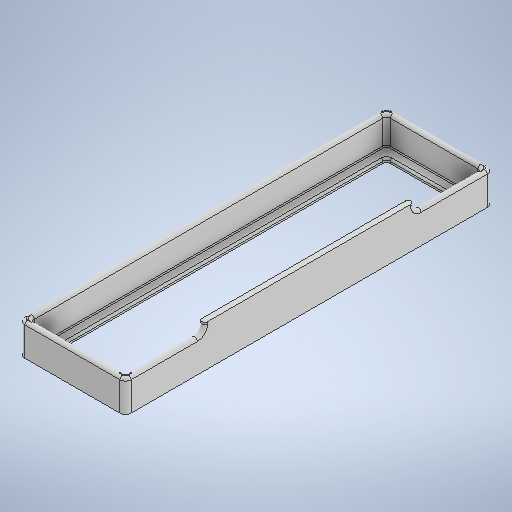
# Autodesk Inventor part: Case for ToolBox
Saved by Autodesk Inventor 2025 (Build 290162000, 162)
## iProperties
Created: 2024-11-06
Part Number: Case for ToolBox
Material: Типовые
Document SubType Name: Modeling
Designer: Makusimu
Density: 1 g/cm^3
Appearance: По умолчанию
Author: Makusimu
Autodesk Inventor part; units mm, degrees
ref_plane "YZ Plane" through (0, 0, 0) normal (1, 0, 0) x (0, 1, 0)
ref_plane "XZ Plane" through (0, 0, 0) normal (0, 1, 0) x (-1, 0, 0)
ref_plane "XY Plane" through (0, 0, 0) normal (0, 0, 1) x (1, 0, 0)
sketch "Эскиз1" plane through (0, 0, 0) normal (0, 1, 0) x (-1, 0, 0)
  line L0 (0, 0) -> (57, 0)
  line L1 (57, 0) -> (57, -197)
  line L2 (57, -197) -> (0, -197)
  line L3 (0, -197) -> (0, 0)
  line L4 (48.5, -8.5) -> (8.5, -8.5)
  line L5 (8.5, -8.5) -> (8.5, -188.5)
  line L6 (8.5, -188.5) -> (48.5, -188.5)
  line L7 (48.5, -188.5) -> (48.5, -8.5)
  point P0 (48.5, -98.5)
  point P1 (57, -98.5)
  point P2 (28.5, 0)
  point P3 (28.5, -8.5)
  dimension "d0" = 57
  dimension "d1" = 197
  dimension "d2" = 40
  dimension "d3" = 180
  dimension "d4" = 0
  dimension "d5" = 0
  constraints: 16 end point, 4 midpoint, 4 parallel, 2 horizontal, 2 perpendicular
  measures "d0" distance of L1.end L2.end
  measures "d1" distance of L0.end L1.end
  measures "d2" distance of L6.end L5.end
  measures "d3" distance of L5.end L4.end
  measures "d4" vertical distance of point (48.5, -98.5) point (57, -98.5)
  measures "d5" horizontal distance of point (28.5, 0) point (28.5, -8.5)
extrude "Выдавливание1" add sketch "Эскиз1" along normal blind 2
sketch "Эскиз2" plane through (0, 2, 0) normal (0, 1, 0) x (1, 0, 0)
  line L0 (-54, 3) -> (-3, 3)
  line L1 (-3, 3) -> (-3, 194)
  line L2 (-3, 194) -> (-54, 194)
  line L3 (-54, 194) -> (-54, 3)
  line L4 (-57, 197) -> (-57, 0) projected
  line L5 (-57, 0) -> (0, 0) projected
  line L6 (0, 0) -> (0, 197) projected
  line L7 (-57, 0) -> (0, 0)
  line L8 (0, 0) -> (0, 197)
  line L9 (0, 197) -> (-57, 197)
  line L10 (-57, 197) -> (-57, 0)
  point P0 (-57, 98.5)
  point P1 (-54, 98.5)
  point P2 (-28.5, 0)
  point P3 (-28.5, 3)
  dimension "d8" = 51
  dimension "d9" = 191
  dimension "d10" = 0
  dimension "d11" = 0
  constraints: 16 end point, 4 midpoint, 4 parallel, 2 horizontal, 2 perpendicular
  measures "d8" distance of L2.end L1.end
  measures "d9" distance of L1.end L0.end
  measures "d10" vertical distance of point (-57, 98.5) point (-54, 98.5)
  measures "d11" horizontal distance of point (-28.5, 0) point (-28.5, 3)
extrude "Выдавливание2" add sketch "Эскиз2" along normal blind 15
fillet "Сопряжение1" radius 2 4 edges at (-48.5, 1, -188.5) (-8.5, 1, -8.5) (-8.5, 1, -188.5) (-48.5, 1, -8.5)
fillet "Сопряжение2" radius 2 4 edges at (-54, 9.5, -3) (-3, 9.5, -3) (-3, 9.5, -194) (-54, 9.5, -194)
fillet "Сопряжение3" radius 3 4 edges at (0, 8.5, 0) (-57, 8.5, 0) (0, 8.5, -197) (-57, 8.5, -197)
fillet "Сопряжение5" radius 0.5 8 edges at (-3.5858, 2, -193.4142) (-28.5, 2, -194) (-53.4142, 2, -193.4142) (-54, 2, -98.5) (-53.4142, 2, -3.5858) (-28.5, 2, -3) (-3.5858, 2, -3.5858) (-3, 2, -98.5)
fillet "Сопряжение6" radius 1 8 edges at (-9.0858, 2, -9.0858) (-28.5, 2, -8.5) (-47.9142, 2, -9.0858) (-48.5, 2, -98.5) (-47.9142, 2, -187.9142) (-28.5, 2, -188.5) (-9.0858, 2, -187.9142) (-8.5, 2, -98.5)
sketch "Эскиз3" plane through (0, 17, 0) normal (0, 1, 0) x (1, 0, 0)
  line L0 (0, 3) -> (0, 194) projected
  line L1 (-3, 192) -> (-3, 5) projected
  line L2 (0, 154.5) -> (-3, 154.5)
  line L3 (-3, 154.5) -> (-3, 42.5)
  line L4 (-3, 42.5) -> (0, 42.5)
  line L5 (0, 42.5) -> (0, 154.5)
  point P0 (0, 0)
  point P1 (0, 98.5)
  point P2 (-1.5, 154.5)
  point P3 (0, 42.5)
  dimension "d20" = 112
  dimension "d21" = 56
  constraints: 8 end point, 2 midpoint, 2 parallel, 2 point on line, 1 horizontal, 1 perpendicular
  measures "d20" distance of L3.end L2.end
  measures "d21" vertical distance of point (0, 98.5) point (-1.5, 154.5)
extrude "Выдавливание3" add sketch "Эскиз3" along normal blind 5
fillet "Сопряжение7" radius 4 2 edges at (-1.5, 17, -42.5) (-1.5, 17, -154.5)
fillet "Сопряжение8" radius 1.5 26 edges at (-56.1213, 17, -0.8787) (-28.5, 17, 0) (-0.8787, 17, -0.8787) (0, 17, -20.75) (0, 18.1716, -41.3284) (0, 21.5, -42.5) (-56.1213, 17, -196.1213) (-28.5, 17, -197) (-0.8787, 17, -196.1213) (0, 17, -176.25) (0, 18.1716, -155.6716) (0, 21.5, -154.5) (-57, 17, -98.5) (-53.4142, 17, -193.4142) (-28.5, 17, -194) (-3.5858, 17, -193.4142) (-3, 17, -175.25) (-3, 18.1716, -155.6716) (-3, 21.5, -154.5) (-53.4142, 17, -3.5858) (-28.5, 17, -3) (-3.5858, 17, -3.5858) (-3, 17, -21.75) (-3, 18.1716, -41.3284) (-3, 21.5, -42.5) (-54, 17, -98.5)
